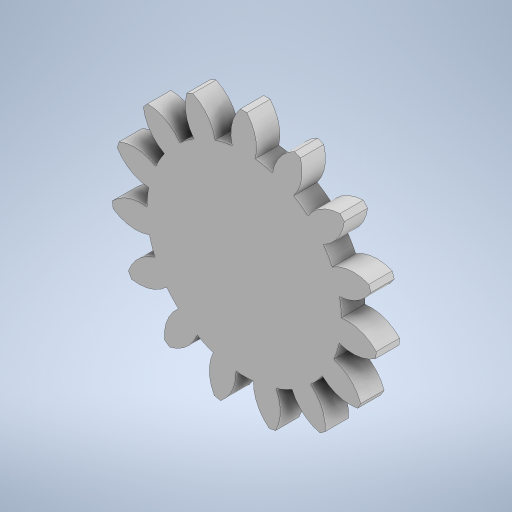
# Autodesk Inventor part: 15P_Recto
Saved by Autodesk Inventor 2023 (Build 270158030, 158C)
## iProperties
Created: 2022-05-28
Part Number: 15P_Recto
Material: Genérico
Document SubType Name: Modeling
Designer: isaac
Density: 1 g/cm^3
Appearance: Valor por defecto
Author: isaac
Autodesk Inventor part; units mm, degrees
ref_plane "YZ Plane" through (0, 0, 0) normal (1, 0, 0) x (0, 1, 0)
ref_plane "XZ Plane" through (0, 0, 0) normal (0, 1, 0) x (-1, 0, 0)
ref_plane "XY Plane" through (0, 0, 0) normal (0, 0, 1) x (1, 0, 0)
sketch "Boceto1" plane through (0, 0, 0) normal (0, 0, 1) x (1, 0, 0)
  arc A0 (168.6959, -21.0168) -> (169.5218, -12.7418) centre (0, 0) ccw
  arc A1 (169.5218, -12.7418) -> (124.9741, 2.5458) centre (132.4533, -48.2091) ccw
  arc A2 (122.0053, -27.1977) -> (168.6959, -21.0168) centre (139.3691, 21.0776) ccw
  arc A3 (162.6596, 49.415) -> (160.0484, 57.3105) centre (0, 0) ccw
  arc A4 (160.0484, 57.3105) -> (113.134, 53.1573) centre (140.6105, 9.8324) ccw
  arc A5 (122.5196, 24.7777) -> (162.6596, 49.415) centre (118.7469, 75.9418) ccw
  arc A6 (128.4981, 111.3025) -> (122.9012, 117.4533) centre (0, 0) ccw
  arc A7 (122.9012, 117.4533) -> (81.7321, 94.5773) centre (124.4549, 66.1738) ccw
  arc A8 (101.8493, 72.4688) -> (128.4981, 111.3025) centre (77.5924, 117.6751) ccw
  arc A9 (72.1181, 153.9447) -> (64.5033, 157.2874) centre (0, 0) ccw
  arc A10 (64.5033, 157.2874) -> (36.1979, 119.6441) centre (86.7799, 111.0732) ccw
  arc A11 (63.5682, 107.6294) -> (72.1181, 153.9447) centre (23.0214, 139.0612) ccw
  arc A12 (3.2682, 169.9686) -> (-5.0479, 169.925) centre (0, 0) ccw
  arc A13 (-5.0479, 169.925) -> (-15.5952, 124.0233) centre (34.0998, 136.767) ccw
  arc A14 (14.2956, 124.1798) -> (3.2682, 169.9686) centre (-35.5302, 136.4024) ccw
  arc A15 (-66.1468, 156.6033) -> (-73.7262, 153.1811) centre (0, 0) ccw
  arc A16 (-73.7262, 153.1811) -> (-64.6918, 106.9578) centre (-24.4764, 138.8125) ccw
  arc A17 (-37.4488, 119.2585) -> (-66.1468, 156.6033) centre (-87.9383, 110.1584) ccw
  arc A18 (-124.1244, 116.1599) -> (-129.6566, 109.9508) centre (0, 0) ccw
  arc A19 (-129.6566, 109.9508) -> (-102.6026, 71.3983) centre (-78.8204, 116.8561) ccw
  arc A20 (-82.718, 93.7163) -> (-124.1244, 116.1599) centre (-125.141, 64.867) ccw
  arc A21 (-160.6398, 55.6314) -> (-163.1682, 47.7089) centre (0, 0) ccw
  arc A22 (-163.1682, 47.7089) -> (-122.7724, 23.4934) centre (-119.5357, 74.6942) ccw
  arc A23 (-113.6845, 51.9696) -> (-160.6398, 55.6314) centre (-140.7058, 8.3595) ccw
  arc A24 (-169.3791, -14.5163) -> (-168.4665, -22.7822) centre (0, 0) ccw
  arc A25 (-168.4665, -22.7822) -> (-121.7138, -28.4738) centre (-139.5821, 19.617) ccw
  arc A26 (-124.9939, 1.237) -> (-169.3791, -14.5163) centre (-131.9412, -49.5935) ccw
  arc A27 (-148.8312, -82.154) -> (-144.6355, -89.3341) centre (0, 0) ccw
  arc A28 (-144.6355, -89.3341) -> (-99.6097, -75.5175) centre (-135.4936, -38.8522) ccw
  arc A29 (-114.6907, -49.7095) -> (-148.8312, -82.154) centre (-100.3628, -98.9712) ccw
  arc A30 (-102.549, -135.5865) -> (-95.7956, -140.4393) centre (0, 0) ccw
  arc A31 (-95.7956, -140.4393) -> (-60.2823, -109.5036) centre (-107.9769, -90.6034) ccw
  arc A32 (-84.5565, -92.0608) -> (-102.549, -135.5865) centre (-51.4308, -131.2359) ccw
  arc A33 (-38.5352, -165.5749) -> (-30.3919, -167.2613) centre (0, 0) ccw
  arc A34 (-30.3919, -167.2613) -> (-10.5315, -124.5556) centre (-61.7901, -126.6885) ccw
  arc A35 (-39.8017, -118.494) -> (-38.5352, -165.5749) centre (6.3941, -140.8088) ccw
  arc A36 (32.1417, -166.9339) -> (40.267, -165.1623) centre (0, 0) ccw
  arc A37 (40.267, -165.1623) -> (41.0403, -118.0707) centre (-4.9192, -140.868) ccw
  arc A38 (11.8352, -124.4385) -> (32.1417, -166.9339) centre (63.1134, -126.0345) ccw
  arc A39 (97.261, -139.4285) -> (103.9632, -134.5052) centre (0, 0) ccw
  arc A40 (103.9632, -134.5052) -> (85.5159, -91.1703) centre (52.8023, -130.6902) ccw
  arc A41 (61.4257, -108.8664) -> (97.261, -139.4285) centre (108.9198, -89.4677) ccw
  arc A42 (145.563, -87.8146) -> (149.6833, -80.5909) centre (0, 0) ccw
  arc A43 (149.6833, -80.5909) -> (115.205, -48.5058) centre (101.3937, -97.9148) ccw
  arc A44 (100.3951, -74.4703) -> (145.563, -87.8146) centre (135.893, -37.4312) ccw
  arc A45 (113.134, 53.1573) -> (101.8493, 72.4688) centre (0, 0) ccw
  arc A46 (124.9741, 2.5458) -> (122.5196, 24.7777) centre (0, 0) ccw
  arc A47 (115.205, -48.5058) -> (122.0053, -27.1977) centre (0, 0) ccw
  arc A48 (85.5159, -91.1703) -> (100.3951, -74.4703) centre (0, 0) ccw
  arc A49 (41.0403, -118.0707) -> (61.4257, -108.8664) centre (0, 0) ccw
  arc A50 (-10.5315, -124.5556) -> (11.8352, -124.4385) centre (0, 0) ccw
  arc A51 (-60.2823, -109.5036) -> (-39.8017, -118.494) centre (0, 0) ccw
  arc A52 (-99.6097, -75.5175) -> (-84.5565, -92.0608) centre (0, 0) ccw
  arc A53 (-121.7138, -28.4738) -> (-114.6907, -49.7095) centre (0, 0) ccw
  arc A54 (-122.7724, 23.4934) -> (-124.9939, 1.237) centre (0, 0) ccw
  arc A55 (-102.6026, 71.3983) -> (-113.6845, 51.9696) centre (0, 0) ccw
  arc A56 (-64.6918, 106.9578) -> (-82.718, 93.7163) centre (0, 0) ccw
  arc A57 (-15.5952, 124.0233) -> (-37.4488, 119.2585) centre (0, 0) ccw
  arc A58 (81.7321, 94.5773) -> (63.5682, 107.6294) centre (0, 0) ccw
  arc A59 (36.1979, 119.6441) -> (14.2956, 124.1798) centre (0, 0) ccw
  dimension "d8" = 360
  constraints: 120 point on circle, 60 centre point, 3 coincident, 149 other
extrude "Extrusión1" add sketch "Boceto1" along normal blind 30
